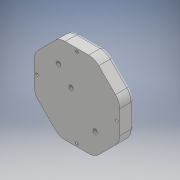
# Autodesk Inventor part: holder
Saved by Autodesk Inventor 2018 (Build 220112000, 112)
## iProperties
Created: 2018-08-13
Part Number: holder
Material: Generic
Document SubType Name: Modeling
Designer: erwin
Density: 1 g/cm^3
Appearance: Default
Author: erwin
Autodesk Inventor part; units mm, degrees
ref_plane "YZ Plane" through (0, 0, 0) normal (1, 0, 0) x (0, 1, 0)
ref_plane "XZ Plane" through (0, 0, 0) normal (0, 1, 0) x (-1, 0, 0)
ref_plane "XY Plane" through (0, 0, 0) normal (0, 0, 1) x (1, 0, 0)
sketch "Sketch5" plane through (0, 0, 0) normal (0, 1, 0) x (-1, 0, 0)
  line L0 (12.4264, 30) -> (30, 12.4264)
  line L1 (30, 12.4264) -> (30, -12.4264)
  line L2 (30, -12.4264) -> (12.4264, -30)
  line L3 (12.4264, -30) -> (-12.4264, -30)
  line L4 (-12.4264, -30) -> (-30, -12.4264)
  line L5 (-30, -12.4264) -> (-30, 12.4264)
  line L6 (-30, 12.4264) -> (-12.4264, 30)
  line L7 (-12.4264, 30) -> (12.4264, 30)
  point P0 (0, 0)
  dimension "d19" = 60
  constraints: 16 end point, 1 horizontal, 17 other
  measures "d19" distance between parallel lines of L3 L7
extrude "Extrusion3" add sketch "Sketch5" along normal blind 10
sketch "Sketch6" plane through (0, 10, 0) normal (0, 1, 0) x (1, 0, 0)
  circle A0 centre (18, 0) radius 0.9
  line L0 (30, -12.4264) -> (30, 12.4264) projected
  line L1 (30, 0) -> (0, 0) construction
  dimension "d11" = 1.8
  dimension "d20" = 12
  constraints: 2 end point, 1 centre point, 1 horizontal, 1 midpoint, 1 point on line
  measures "d11" diameter of A0
  measures "d20" distance from line of L0 A0.centre
sketch "Sketch8" plane through (30, 0, 12.4264) normal (1, 0, 0) x (0, 0, -1)
  circle A0 centre (12.4264, -2) radius 0.9
  line L0 (0, 10) -> (24.8528, 10) projected
  line L1 (12.4264, 0) -> (12.4264, 10) construction
  dimension "d21" = 1.8
  dimension "d22" = 12
  constraints: 2 end point, 1 centre point, 1 midpoint, 1 point on line
  measures "d21" diameter of A0
  measures "d22" distance from line of L0 A0.centre
loft "Loft2" cut profiles "Sketch8", "Sketch6"
pattern_circular "Circular Pattern1" count 4 over 360 about axis through (0, -10, 0) along (0, 1, 0) of "Loft2"
sketch "Sketch9" plane through (0, 10, 0) normal (0, 1, 0) x (1, 0, 0)
  line L0 (-5.3033, 8.8388) -> (8.8388, -5.3033)
  line L1 (8.8388, -5.3033) -> (5.3033, -8.8388)
  line L2 (5.3033, -8.8388) -> (-8.8388, 5.3033)
  line L3 (-8.8388, 5.3033) -> (-5.3033, 8.8388)
  line L4 (-5.3033, 8.8388) -> (5.3033, -8.8388) construction
  line L5 (8.8388, -5.3033) -> (-8.8388, 5.3033) construction
  line L6 (-30, -12.4264) -> (-12.4264, -30) construction
  point P0 (0, 0)
  dimension "d30" = 5
  dimension "d62" = 20
  constraints: 12 end point, 3 parallel, 2 midpoint, 1 perpendicular
  measures "d30" distance between parallel lines of L0 L2
  measures "d62" distance of L0.start L0.end
extrude "Extrusion4" add sketch "Sketch9" along normal blind 10
sketch "Sketch10" plane through (0, 20, 0) normal (0, 1, 0) x (1, 0, 0)
  point P0 (0, 0)
  point P1 (0, 0)
  constraints: 1 coincident
hole "Hole1" at (0, 20, 0) direction (0, -1, 0) diameter 1.8 depth 15 tip angle 118
chamfer "Chamfer1" distance 5 angle 45 2 edges at (7.0711, 20, 7.0711) (-7.0711, 20, -7.0711)
fillet "Fillet3" radius 10 8 edges at (-30, 5, 12.4264) (-12.4264, 5, 30) (-30, 5, -12.4264) (-12.4264, 5, -30) (12.4264, 5, 30) (12.4264, 5, -30) (30, 5, -12.4264) (30, 5, 12.4264)
fillet "Fillet3" radius 2 10 edges at (21.2132, 10, -21.2132) (0, 10, -30) (30, 10, 0) (-30, 10, 0) (-21.2132, 10, 21.2132) (0, 10, 30) (-21.2132, 10, -21.2132) (21.2132, 10, 21.2132) (-7.0711, 10, -7.0711) (7.0711, 10, 7.0711)
fillet "Fillet3" radius 4 4 edges at (-7.0711, 15, -7.0711) (-3.5355, 20, -3.5355) (3.5355, 20, 3.5355) (7.0711, 15, 7.0711)
sketch "Sketch12" plane through (0, 10, 0) normal (0, -1, 0) x (1, 0, 0)
  line L0 (17.3636, -0.6364) -> (-0.6364, -18.6364) construction
  line L1 (12.8636, -5.1364) -> (3.8636, -5.1364) construction
  line L2 (3.8636, -5.1364) -> (3.8636, -14.1364) construction
  line L3 (3.8636, -14.1364) -> (12.8636, -14.1364) construction
  line L4 (12.8636, -14.1364) -> (12.8636, -5.1364) construction
  line L5 (12.8636, -5.1364) -> (3.8636, -14.1364) construction
  line L6 (3.8636, -5.1364) -> (12.8636, -14.1364) construction
  point P0 (0, 0)
  point P1 (18.9, 0)
  point P2 (0, -18.9)
  point P3 (8.3636, -9.6364)
  dimension "d51" = 9
  constraints: 14 end point, 3 midpoint, 2 parallel, 1 coincident, 1 horizontal, 1 perpendicular, 1 point on line, 6 other
  measures "d51" distance of L2.end L3.end
hole "Hole2" at (12.8636, 10, -14.1364) direction (0, -1, 0) diameter 3 end through all counterbore diameter 5 counterbore depth 1
pattern_circular "Circular Pattern2" count 2 over 360 about axis through (0, 12.5, 0) along (0, 1, 0) of "Hole2"
sketch "Sketch14" plane through (-8.8388, 10, -5.3033) normal (-0.7071, 0, 0.7071) x (0.7071, 0, 0.7071)
  line L0 (9.4021, 23.2185) -> (10.4021, 23.2185)
  line L1 (10.4021, 23.2185) -> (10.4021, 1)
  line L2 (10.4021, 1) -> (9.4021, 1)
  line L3 (9.4021, 1) -> (9.4021, 23.2185)
  line L4 (9.4021, 23.2185) -> (10.4021, 1) construction
  line L5 (10.4021, 23.2185) -> (9.4021, 1) construction
  line L6 (18.2843, 0) -> (1.7157, 0) projected
  point P0 (10, -10)
  point P1 (9.9021, 12.1093)
  dimension "d63" = 1
  dimension "d64" = 1
  constraints: 12 end point, 2 midpoint, 2 parallel, 1 horizontal, 1 perpendicular
  measures "d63" distance of L1.end L2.end
  measures "d64" distance from line of L6 L2.end
extrude "Extrusion6" cut sketch "Sketch14" against normal up to surface
sketch "Sketch15" plane through (0, 10, 0) normal (0, 1, 0) x (1, 0, 0)
  line L0 (0, 0) -> (-4, -4) construction
  line L1 (8.2843, -28) -> (-8.2843, -28) construction
  point P0 (14.2843, -28)
  dimension "d67" = 45
  dimension "d68" = 4
  constraints: 2 end point
  measures "d67" angle of L1 L0
  measures "d68" horizontal distance of L0.start L0.end
hole "Hole3" at (-4, 10, 4) direction (0, -1, 0) diameter 3 end through all
equation "\"d22\" = d20"
body "Solid2"
